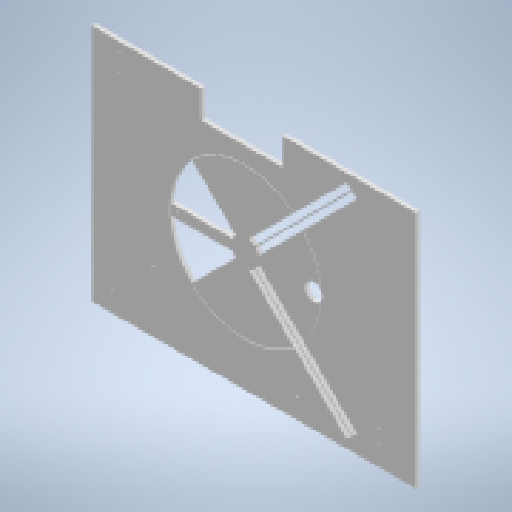
# Autodesk Inventor part: Wheel1
Saved by Autodesk Inventor 2023 (Build 270158000, 158)
## iProperties
Created: 2023-05-10
Part Number: Wheel1
Material: Generic
Document SubType Name: Modeling
Designer: Nathann
Density: 1 g/cm^3
Appearance: Default
Author: Nathann
Autodesk Inventor part; units mm, degrees
ref_plane "YZ Plane" through (0, 0, 0) normal (1, 0, 0) x (0, 1, 0)
ref_plane "XZ Plane" through (0, 0, 0) normal (0, 1, 0) x (-1, 0, 0)
ref_plane "XY Plane" through (0, 0, 0) normal (0, 0, 1) x (1, 0, 0)
sketch "Sketch1" plane through (0, 0, 0) normal (0, 0, 1) x (1, 0, 0)
  line L0 (0, 0) -> (-400, 0)
  line L1 (-400, 0) -> (-400, 350)
  line L2 (-400, 350) -> (0, 350)
  line L3 (0, 350) -> (0, 0)
  circle A0 centre (-175, 175) radius 110
  circle A1 centre (-175, 175) radius 20
  line L4 (-160.8579, 160.8579) -> (0, 0)
  line L5 (0, 350) -> (-160.8579, 189.1421)
  line L6 (-169.8236, 194.3185) -> (-26.5076, 337.6346)
  line L7 (-26.5076, 337.6346) -> (-12.3654, 323.4924)
  line L8 (-12.3654, 323.4924) -> (-155.6815, 180.1764)
  line L9 (-155.6815, 169.8236) -> (-12.1198, 26.262)
  line L10 (-169.8236, 155.6815) -> (-26.7532, 12.6111)
  line L11 (-26.7532, 12.6111) -> (-12.1198, 26.262)
  line L12 (-160.1684, 188.4173) -> (-18.7294, 329.8564)
  line L13 (-20.1436, 331.2706) -> (-161.5827, 189.8316)
  line L14 (-160.1684, 161.5827) -> (-18.7048, 20.1191)
  line L15 (-20.1682, 18.754) -> (-161.5827, 160.1684)
  circle A2 centre (-175, 175) radius 111
  line L16 (-400, 0) -> (-317.8714, 0)
  line L17 (-317.8714, 0) -> (-317.8714, 55)
  line L18 (-317.8714, 55) -> (-400, 55)
  line L19 (-400, 55) -> (-400, 0)
  line L20 (-317.8714, 0) -> (-307.8714, 0)
  line L21 (-307.8714, 0) -> (-307.8714, 155)
  line L22 (-317.8714, 155) -> (-317.8714, 0)
  line L23 (-317.8714, 55) -> (-320.1214, 55)
  line L24 (-320.1214, 55) -> (-320.1214, 155)
  line L25 (-320.1214, 155) -> (-317.8714, 155)
  line L26 (-317.8714, 155) -> (-317.8714, 55)
  line L27 (-400, 55) -> (-397.75, 55)
  line L28 (-397.75, 55) -> (-397.75, 155)
  line L29 (-397.75, 155) -> (-400, 155)
  line L30 (-400, 155) -> (-400, 55)
  line L31 (-400, 155) -> (-307.8714, 155)
  line L32 (-307.8714, 155) -> (-307.8714, 175)
  line L33 (-307.8714, 175) -> (-400, 175)
  line L34 (-400, 175) -> (-400, 155)
  line L35 (-175, 175) -> (-307.8714, 175)
  line L36 (-307.8714, 175) -> (-307.8714, 171)
  line L37 (-307.8714, 171) -> (-175, 171)
  line L38 (-175, 171) -> (-175, 175)
  line L39 (-307.8714, 169) -> (-175, 169)
  line L40 (-175, 169) -> (-175, 165)
  line L41 (-175, 165) -> (-307.8714, 165)
  line L42 (-307.8714, 165) -> (-307.8714, 169)
  line L43 (-317.8714, 155) -> (-297.8714, 155)
  line L44 (-297.8714, 155) -> (-297.8714, 165)
  line L45 (-297.8714, 165) -> (-317.8714, 165)
  line L46 (-317.8714, 165) -> (-317.8714, 155)
  line L47 (-400, 175) -> (-285.6082, 175)
  line L48 (-285.6082, 175) -> (-285.6082, 179.6746)
  line L49 (-285.6082, 179.6746) -> (-400, 179.6746)
  line L50 (-400, 179.6746) -> (-400, 175)
  point P0 (-19.4365, 330.5635)
  point P1 (-19.4365, 19.4365)
  point P2 (-89.7592, 246.0986)
  point P3 (-89.7592, 103.9014)
  point P4 (-90.4693, 104.6114)
  point P5 (-90.4693, 245.3886)
  point P6 (-104.6114, 259.5307)
  point P7 (-104.6114, 90.4693)
  point P8 (-103.9014, 89.7592)
  point P9 (-103.9014, 260.2408)
  point P10 (-317.8714, 27.5)
  point P11 (-285.5486, 165)
  point P12 (-284.5445, 165)
  point P13 (-317.8714, 0)
  point P14 (-285, 175)
  point P15 (-286, 175)
  point P16 (-285.8377, 169)
  point P17 (-194.0788, 169)
  point P18 (-192.3205, 165)
  point P19 (-97.9286, 96.5144)
  point P20 (-97.2214, 95.8072)
  point P21 (-284.8362, 169)
  point P22 (-96.5144, 97.9286)
  point P23 (-96.5144, 252.0714)
  point P24 (-97.9286, 253.4856)
  point P25 (-97.2214, 254.1928)
  point P26 (-95.8072, 252.7786)
  point P27 (-95.8072, 97.2214)
  point P28 (-285.9015, 179.6746)
  dimension "d7" = 40
  dimension "d0" = 350
  dimension "d1" = 400
  dimension "d4" = 175
  dimension "d5" = 175
  dimension "d6" = 220
  dimension "d8" = 10
  dimension "d9" = 10
  dimension "d10" = 10
  dimension "d11" = 10
  dimension "d12" = 1
  dimension "d13" = 1
  dimension "d14" = 1
  dimension "d15" = 1
  dimension "d16" = 200
  dimension "d17" = 200
  dimension "d18" = 222
  dimension "d19" = 100
  dimension "d20" = 2.25
  dimension "d21" = 2.25
  dimension "d22" = 10
  dimension "d24" = 20
  dimension "d25" = 0
  dimension "d26" = 6
  dimension "d27" = 4
  dimension "d28" = 4
  dimension "d29" = 20
  dimension "d30" = 0
  constraints: 102 end point, 25 parallel, 12 perpendicular, 11 point on line, 10 horizontal, 3 midpoint, 2 centre point, 2 coincident, 12 other
  measures "d0" distance of L2.end L0.start
  measures "d1" distance of L0.start L0.end
  measures "d4" distance from line of L3 A0.centre
  measures "d5" distance from line of L0 A0.centre
  measures "d6" diameter of A0
  measures "d8" distance between parallel lines of L6 L5
  measures "d9" distance between parallel lines of L8 L5
  measures "d10" distance between parallel lines of L9 L4
  measures "d11" distance between parallel lines of L4 L10
  measures "d12" distance between parallel lines of L13 L5
  measures "d13" distance between parallel lines of L12 L5
  measures "d14" distance between parallel lines of L14 L4
  measures "d15" distance between parallel lines of L15 L4
  measures "d16" distance of point (-19.437, 330.563) L5.end
  measures "d17" distance of point (-19.437, 19.437) L4.start
  measures "d18" diameter of A2
  measures "d19" distance between parallel lines of L18 L31
  measures "d20" distance between parallel lines of L24 L26
  measures "d21" distance between parallel lines of L1 L28
  measures "d22" distance from line of point (-317.871, 27.5) L21
  measures "d24" distance between parallel lines of L31 L33
  measures "d25" distance from line of L33 point (-175, 175)
  measures "d26" distance from line of L39 A0.centre
  measures "d27" distance between parallel lines of L41 L39
  measures "d28" distance between parallel lines of L35 L37
  measures "d29" distance between parallel lines of L46 L44
  measures "d30" distance from line of point (-175, 175) L35
extrude "Extrusion1" add sketch "Sketch1" along normal blind 6 contours L4 L11 L9 A2 L8 L7 L5 L3 | L0 L21 L43 L44 L41 A2 L10 L11 L4 | L0 L17 L22 L31 L21 | L5 L7 L6 A2 L49 L1 L2 | L11 L15 A2 L4 | L4 A2 L14 L11 | L0 L1 L18 L17 | L31 L46 L45 L32 | L32 L41 L44 L43 | L7 L12 A2 L5 | L5 A2 L13 L7 | A2 L15 A0 L4 | L4 A0 L14 A2 | L18 L24 L25 L22 | L25 L31 L29 L1 L33 L32 L45 L46 | L32 L39 A2 L41 | L49 A2 L35 L33 L1 | A2 L12 A0 L5 | L5 A0 L13 A2 | L4 A1 L14 A0 | A0 L15 A1 L4 | L1 L29 L28 L18 | L18 L28 L31 L24 | L32 L37 A2 L39 | L5 A1 L13 A0 | A0 L12 A1 L5 | A1 L41 L40 L39 L37 L38 L35 | L32 L35 A2 L37 | A0 L41 A1 L10 | L9 A1 L8 A0 | L39 A1 L41 A0 | A0 L37 A1 L39 | L6 A1 L35 A0 | A0 L35 A1 L37 | L39 L40 L41 A1 | A1 L35 L38 L37
sketch "Sketch2" plane through (0, 0, 0) normal (0, 0, -1) x (-1, 0, 0)
  arc A0 (285.9015, 179.6746) -> (103.9014, 260.2408) centre (175, 175) ccw projected
  circle A1 centre (275, 175) radius 1.5
  circle A2 centre (75, 175) radius 12.5
  point P0 (0, 0)
  dimension "d31" = 3
  dimension "d32" = 0
  dimension "d33" = 100
  dimension "d36" = 100
  dimension "d37" = 25
  constraints: 2 centre point
  measures "d31" diameter of A1
  measures "d32" vertical distance of A1.centre A0.centre
  measures "d33" distance of A1.centre A0.centre
  measures "d36" distance of A2.centre A0.centre
  measures "d37" diameter of A2
extrude "Extrusion2" cut sketch "Sketch2" against normal blind 6
sketch "Sketch3" plane through (0, 0, 6) normal (0, 0, 1) x (1, 0, 0)
  line L0 (0, 350) -> (-400, 350) projected
  line L1 (-120, 350) -> (-240, 350)
  line L2 (-240, 350) -> (-240, 310)
  line L3 (-240, 310) -> (-120, 310)
  line L4 (-120, 310) -> (-120, 350)
  line L5 (0, 0) -> (0, 350) projected
  dimension "d40" = 40
  dimension "d41" = 120
  dimension "d42" = 120
  constraints: 8 end point, 2 parallel, 1 horizontal, 1 perpendicular, 1 point on line
  measures "d40" distance of L3.end L1.start
  measures "d41" distance of L2.end L3.end
  measures "d42" distance between parallel lines of L5 L4
extrude "Extrusion3" cut sketch "Sketch3" against normal blind 6
sketch "Sketch4" plane through (0, 0, 6) normal (0, 0, 1) x (1, 0, 0)
  line L0 (-240, 310) -> (-240, 350) projected
  line L1 (-307.8714, 350) -> (-240, 350) projected
  line L2 (-307.8714, 341) -> (-307.8714, 350) projected
  line L3 (-275, 341) -> (-307.8714, 341) projected
  line L4 (-275, 309) -> (-275, 341) projected
  line L5 (-307.8714, 309) -> (-275, 309) projected
  line L6 (-307.8714, 195) -> (-307.8714, 309) projected
  line L7 (-297.8714, 195) -> (-307.8714, 195) projected
  line L8 (-297.8714, 185) -> (-297.8714, 195) projected
  line L9 (-285.5486, 185) -> (-297.8714, 185) projected
  line L10 (-26.7532, 337.3889) -> (-103.9014, 260.2408) projected
  line L11 (-20.1682, 331.246) -> (-26.7532, 337.3889) projected
  line L12 (-161.5827, 189.8316) -> (-20.1682, 331.246) projected
  line L13 (-104.6114, 259.5307) -> (-169.8236, 194.3185) projected
  line L14 (-175, 185) -> (-284.5445, 185) projected
  line L15 (-175, 181) -> (-175, 185) projected
  line L16 (-307.8714, 181) -> (-175, 181) projected
  line L17 (-307.8714, 185) -> (-307.8714, 181) projected
  line L18 (-317.8714, 185) -> (-307.8714, 185) projected
  line L19 (-317.8714, 310) -> (-317.8714, 185) projected
  line L20 (-285, 310) -> (-317.8714, 310) projected
  line L21 (-285, 340) -> (-285, 310) projected
  line L22 (-317.8714, 340) -> (-285, 340) projected
  line L23 (-317.8714, 350) -> (-317.8714, 340) projected
  line L24 (-400, 350) -> (-317.8714, 350) projected
  line L25 (-400, 175) -> (-400, 350) projected
  line L26 (-307.8714, 175) -> (-400, 175) projected
  line L27 (-307.8714, 179) -> (-307.8714, 175) projected
  line L28 (-175, 179) -> (-307.8714, 179) projected
  line L29 (-175, 175) -> (-175, 179) projected
  line L30 (-262.5741, 175) -> (-175, 175) projected
  line L31 (-169.8236, 155.6815) -> (-104.6114, 90.4693) projected
  line L32 (-20.1436, 18.7294) -> (-161.5827, 160.1684) projected
  line L33 (-26.5076, 12.3654) -> (-20.1436, 18.7294) projected
  line L34 (-103.9014, 89.7592) -> (-26.5076, 12.3654) projected
  line L35 (-400, 170.3254) -> (-286.7025, 170.3254) projected
  line L36 (-400, 0) -> (-400, 170.3254) projected
  line L37 (-120, 350) -> (-120, 310) projected
  line L38 (-120, 310) -> (-240, 310) projected
  line L39 (-160.1684, 161.5827) -> (-18.7294, 20.1436) projected
  line L40 (-12.3654, 26.5076) -> (-89.7592, 103.9014) projected
  line L41 (-155.6815, 180.1764) -> (-143.7852, 192.0727) projected
  line L42 (-18.7048, 329.8809) -> (-160.1684, 188.4173) projected
  line L43 (-12.1198, 323.738) -> (-18.7048, 329.8809) projected
  line L44 (-89.7592, 246.0986) -> (-12.1198, 323.738) projected
  line L45 (-18.7294, 20.1436) -> (-12.3654, 26.5076) projected
  line L46 (-397.75, 195) -> (-320.1214, 195) projected
  line L47 (-397.75, 295) -> (-397.75, 195) projected
  line L48 (-320.1214, 295) -> (-397.75, 295) projected
  line L49 (-320.1214, 195) -> (-320.1214, 295) projected
  circle A0 centre (-100, 30) radius 1.5 projected
  circle A1 centre (-310, 90) radius 1.5 projected
  circle A2 centre (-370, 30) radius 1.5 projected
  arc A3 (-103.9014, 260.2408) -> (-285.5486, 185) centre (-175, 175) ccw projected
  arc A4 (-161.5827, 189.8316) -> (-169.8236, 194.3185) centre (-175, 175) ccw projected
  arc A5 (-104.6114, 259.5307) -> (-284.5445, 185) centre (-175, 175) ccw projected
  arc A6 (-284.7044, 166.9419) -> (-262.5741, 175) centre (-275.0738, 174.9106) ccw projected
  arc A7 (-284.7044, 166.9419) -> (-104.6114, 90.4693) centre (-175, 175) ccw projected
  arc A8 (-169.8236, 155.6815) -> (-161.5827, 160.1684) centre (-175, 175) ccw projected
  arc A9 (-285.81, 168.5087) -> (-103.9014, 89.7592) centre (-175, 175) ccw projected
  arc A10 (-286.7025, 170.3254) -> (-285.81, 168.5087) centre (-275.0738, 174.9106) ccw projected
  arc A11 (-160.1684, 161.5827) -> (-155.6815, 169.8236) centre (-175, 175) ccw projected
  arc A12 (-65.2913, 167) -> (-65.2913, 183) centre (-175, 175) ccw projected
  arc A13 (-155.6815, 180.1764) -> (-160.1684, 188.4173) centre (-175, 175) ccw projected
  arc A14 (-89.7592, 103.9014) -> (-89.7592, 246.0986) centre (-175, 175) ccw projected
  circle A15 centre (-75, 175) radius 1.5 projected
  line L50 (-143.7852, 157.9273) -> (-143.7852, 167) projected
  line L51 (-143.7852, 167) -> (-65.2913, 167) projected
  line L52 (-65.2913, 183) -> (-143.7852, 183) projected
  line L53 (-143.7852, 183) -> (-143.7852, 192.0727) projected
  line L54 (-143.7852, 157.9273) -> (-155.6815, 169.8236) projected
  arc A16 (-332.8714, 308.5) -> (-332.8714, 311.5) centre (-332.8714, 310) ccw projected
  line L55 (-332.8714, 308.5) -> (-385, 308.5) projected
  arc A17 (-385, 311.5) -> (-385, 308.5) centre (-385, 310) ccw projected
  line L56 (-385, 311.5) -> (-332.8714, 311.5) projected
  line L57 (-332.8714, 333.5) -> (-385, 333.5) projected
  arc A18 (-385, 336.5) -> (-385, 333.5) centre (-385, 335) ccw projected
  line L58 (-385, 336.5) -> (-332.8714, 336.5) projected
  arc A19 (-332.8714, 333.5) -> (-332.8714, 336.5) centre (-332.8714, 335) ccw projected
  line L59 (-400, 0) -> (75, 0) projected
  line L60 (75, 0) -> (75, 350) projected
  line L61 (-120, 350) -> (75, 350) projected
  arc A20 (20.1179, 28.5046) -> (19.8821, 28.5046) centre (20, 30) ccw projected
  line L62 (20.1179, 28.5046) -> (19.8821, 28.5046) projected
  circle A21 centre (20, 50) radius 1.5 projected
  point P0 (0, 0)
extrude "Extrusion4" cut sketch "Sketch4" against normal blind 6 contours A0 | A1 | A2
sketch "Sketch5" plane through (0, 0, 6) normal (0, 0, 1) x (1, 0, 0)
  circle A0 centre (-275, 175) radius 1.5 projected
  arc A1 (-104.6114, 259.5307) -> (-104.6114, 90.4693) centre (-175, 175) ccw projected
  line L0 (-284.7087, 167) -> (-193.3303, 167)
  arc A2 (-103.9014, 260.2408) -> (-103.9014, 89.7592) centre (-175, 175) ccw projected
  line L1 (-284.7087, 183) -> (-193.3303, 183)
  arc A3 (-169.8236, 155.6815) -> (-161.5827, 160.1684) centre (-175, 175) ccw projected
  arc A4 (-169.8236, 155.6815) -> (-161.5827, 160.1684) centre (-175, 175) ccw projected
  circle A5 centre (-175, 175) radius 20
  line L2 (-175, 175) -> (-252.7817, 97.2183)
  line L3 (-175, 175) -> (-252.7817, 252.7817)
  point P0 (0, 0)
  point P1 (-189.1421, 189.1421)
  point P2 (-189.1421, 160.8579)
  dimension "d45" = 8
  dimension "d46" = 8
  dimension "d47" = 45
  dimension "d48" = 45
  constraints: 8 end point, 7 point on circle, 2 horizontal, 1 centre point, 1 coincident
  measures "d45" distance from line of L1 A0.centre
  measures "d46" distance from line of L0 A0.centre
  measures "d47" angle of L1 L3
  measures "d48" angle of L2 L0
extrude "Extrusion5" cut sketch "Sketch5" against normal blind 10 contours L3 A5 L1 A1 | L0 A5 L2 A1
sketch "Sketch6" plane through (0, 0, 6) normal (0, 0, 1) x (1, 0, 0)
  circle A0 centre (-360, 335) radius 1.5
  circle A1 centre (-360, 310) radius 1.5
  line L0 (-240, 350) -> (-400, 350) projected
  line L1 (-400, 350) -> (-400, 0) projected
  point P0 (0, 0)
  dimension "d51" = 3
  dimension "d52" = 15
  dimension "d53" = 25
  dimension "d54" = 3
  dimension "d55" = 40
  dimension "d56" = 40
  constraints: 2 centre point
  measures "d51" diameter of A0
  measures "d52" distance from line of L0 A0.centre
  measures "d53" distance of A1.centre A0.centre
  measures "d54" diameter of A1
  measures "d55" distance from line of L1 A0.centre
  measures "d56" distance from line of L1 A1.centre
extrude "Extrusion6" cut sketch "Sketch6" against normal blind 10
sketch "Sketch7" plane through (0, 0, 6) normal (0, 0, 1) x (1, 0, 0)
  line L0 (0, 0) -> (0, 350) projected
  line L1 (0, 0) -> (75, 0)
  line L2 (75, 0) -> (75, 350)
  line L3 (75, 350) -> (0, 350)
  line L4 (0, 350) -> (0, 0)
  line L5 (-400, 350) -> (-400, 0) projected
  point P0 (75, 175)
  dimension "d59" = 475
  constraints: 8 end point, 2 parallel, 1 horizontal, 1 midpoint, 1 perpendicular
  measures "d59" distance from line of point (75, 175) L5
extrude "Extrusion7" add sketch "Sketch7" against normal blind 6
sketch "Sketch8" plane through (0, 0, 0) normal (0, 0, -1) x (-1, 0, 0)
  circle A0 centre (-20, 50) radius 1.5 projected
  arc A1 (-19.8821, 28.5046) -> (-20.1179, 28.5046) centre (-20, 30) ccw projected
  circle A2 centre (-20, 30) radius 1.5
  point P0 (0, 0)
  point P1 (-20.1179, 28.5046)
  point P2 (-19.8821, 28.5046)
  constraints: 1 centre point, 1 coincident, 1 concentric
extrude "Extrusion8" cut sketch "Sketch8" against normal blind 6
equation "\"d4\" = d5"
equation "\"d5\" = 0.5 * d0"
equation "\"d13\" = d12"
equation "\"d15\" = d14"
equation "\"d16\" = BladeLengthRCC"
equation "\"d17\" = d16"
equation "\"d19\" = bladeLengthZeroConverter"
equation "\"d20\" = bladeThicknessZeroConverter"
equation "\"d21\" = bladeThicknessZeroConverter"
equation "\"d27\" = d28"
equation "\"d2\" = thicknessWheelPlate"
equation "\"d34\" = thicknessWheelPlate"
equation "\"d38\" = thicknessWheelPlate"
equation "\"d43\" = thicknessWheelPlate"
equation "\"d56\" = d55"
equation "\"bladeThicknessTablePushing\" = 1"
equation "\"bladeThicknessTable\" = 1"
equation "\"bladeThicknessForceConverter\" = 2"
equation "\"bladeThicknessWheelAnchor\" = 1"
equation "\"BladeThicknessRCC\" = 1"
equation "\"bladeThicknessZeroConverter\" = 2.25"
equation "\"rangeXProbeMax\" = 1"
equation "\"rangeXProbeMin\" = -1"
equation "\"BladeLengthRCC\" = 200"
equation "\"bladeLengthZeroConverter\" = 100"
equation "\"safetyPlay\" = 0.1"
equation "\"OffsetMotorSpring\" = -1"
equation "\"thicknessWheelPlate\" = 6"
equation "\"thicknessConverterPlate\" = 6"
body "Solid1"
